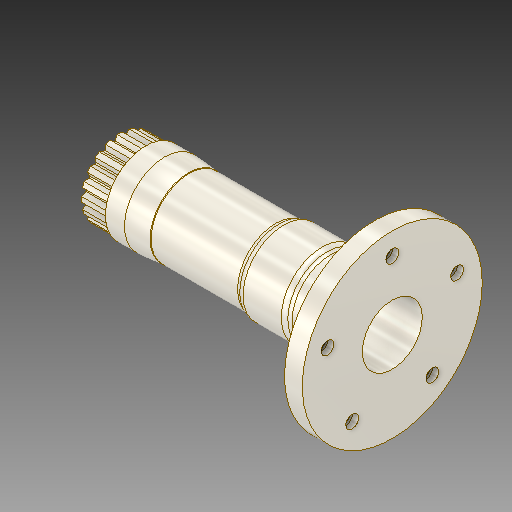
# Autodesk Inventor part: 301-04
Saved by Autodesk Inventor 2019 (Build 230136000, 136)
## iProperties
Company: Autodesk Inc.
Created: 2017-03-16
Part Number: 301-04
Material: Titanium
Document SubType Name: Modeling
Designer: Autodesk Inc.
Density: 4.51 g/cm^3
Appearance: Titanium
Mass: 190.026 g
Surface Area: 234.594 cm^2
Volume: 42.1344 cm^3
Author: Inventor
Autodesk Inventor part; units mm, degrees
ref_plane "YZ Plane" through (0, 0, 0) normal (1, 0, 0) x (0, 1, 0)
ref_plane "XZ Plane" through (0, 0, 0) normal (0, 1, 0) x (-1, 0, 0)
ref_plane "XY Plane" through (0, 0, 0) normal (0, 0, 1) x (1, 0, 0)
sketch "Sketch1" plane through (0, 0, 0) normal (0, 0, 1) x (1, 0, 0)
  line L0 (-20, 0) -> (120, 0) projected
  line L1 (0, 11) -> (100, 11)
  line L2 (0, 11) -> (0, 14.75)
  line L3 (0, 14.75) -> (16.5, 14.75)
  line L4 (58, 15) -> (76.5, 15)
  line L5 (76.5, 15) -> (76.5, 14)
  line L6 (25.3424, 14) -> (58, 14)
  line L7 (100, 14) -> (100, 11)
  line L8 (58, 14) -> (58, 15)
  line L9 (76.5, 14) -> (100, 14)
  arc A0 (25.3424, 14) -> (16.5, 14.75) centre (16.5, -37.75) ccw
  point P0 (0, 0)
  dimension "d0" = 100
  dimension "d1" = 22
  dimension "d2" = 3.75
  dimension "d3" = 16.5
  dimension "d9" = 3
  dimension "d10" = 52.5
  dimension "d11" = 58
  dimension "d12" = 18.5
  dimension "d13" = 4
  constraints: 18 end point, 4 parallel, 3 perpendicular, 2 point on circle, 2 vertical, 1 centre point, 1 collinear, 1 horizontal, 1 point on line, 1 tangent
  measures "d0" distance of L1.start L1.end
  measures "d1" diameter of L1 L0
  measures "d2" distance of L1.start L2.end
  measures "d3" distance of L2.end L3.end
  measures "d9" distance between parallel lines of L1 L6
  measures "d10" radius of A0
  measures "d11" distance between parallel lines of L2 L8
  measures "d12" distance between parallel lines of L8 L5
  measures "d13" distance between parallel lines of L1 L4
revolve "Revolution1" add sketch "Sketch1" angle 360 about axis through (-10, 0, 0) along (1, 0, 0)
fillet "Fillet1" radius 3 2 edges at (58, -15, 0) (76.5, -15, 0)
sketch "Sketch2" plane through (100, 0, 0) normal (1, 0, 0) x (0, 0, -1)
  circle A0 centre (0, 0) radius 14 projected
  circle A1 centre (0, 0) radius 11 projected
  circle A2 centre (0, 0) radius 33
  dimension "d17" = 66
  constraints: 1 centre point, 1 coincident
  measures "d17" diameter of A2
extrude "Extrusion1" add sketch "Sketch2" against normal blind 6.5 contours A2
fillet "Fillet2" radius 2 4 edges at (25.3424, -14, 0) (58, -14, 0) (76.5, -14, 0) (93.5, -14, 0)
ref_plane "Work Plane1" through (94.55, 0, 0) normal (-1, 0, 0) x (0, 0, 1)
sketch "Sketch3" plane through (94.55, 0, 0) normal (-1, 0, 0) x (0, 0, 1)
  circle A0 centre (0, 0) radius 33 projected
  point P0 (0, 25)
  dimension "d20" = 25
  constraints: 1 vertical alignment
  measures "d20" distance of A0.centre point (0, 25)
hole "Hole1" at (94.55, 25, 0) direction (1, 0, 0) diameter 6 depth 5 tip angle 110 start extended yes countersink diameter 11.4 countersink angle 90
pattern_circular "Circular Pattern1" count 5 over 360 about axis through (-10, 0, 0) along (1, 0, 0) of "Hole1"
sketch "Sketch4" plane through (0, 0, 0) normal (-1, 0, 0) x (0, 0, 1)
  circle A0 centre (0, 0) radius 11 projected
  circle A1 centre (0, 0) radius 14.75 projected
  arc A2 (-5.4322, 11.258) -> (-5.9149, 11.012) centre (0, 0) ccw
  line L0 (0, -21) -> (0, 21) construction
  line L1 (-0.9, 14) -> (0.9, 14)
  line L2 (-0.9, 14) -> (-1.6874, 12.3856)
  line L3 (0.9, 14) -> (1.6874, 12.3856)
  line L4 (-5.1822, 13.0367) -> (-5.4322, 11.258)
  line L5 (-5.1822, 13.0367) -> (-3.4703, 13.5929)
  line L6 (-3.4703, 13.5929) -> (-2.2225, 12.3008)
  line L7 (-8.9571, 10.7972) -> (-8.6452, 9.0283)
  line L8 (-8.9571, 10.7972) -> (-7.5009, 11.8552)
  line L9 (-7.5009, 11.8552) -> (-5.9149, 11.012)
  line L10 (-11.8552, 7.5009) -> (-11.012, 5.9149)
  line L11 (-11.8552, 7.5009) -> (-10.7972, 8.9571)
  line L12 (-10.7972, 8.9571) -> (-9.0283, 8.6452)
  line L13 (-13.5929, 3.4703) -> (-12.3008, 2.2225)
  line L14 (-13.5929, 3.4703) -> (-13.0367, 5.1822)
  line L15 (-13.0367, 5.1822) -> (-11.258, 5.4322)
  line L16 (-14, -0.9) -> (-12.3856, -1.6874)
  line L17 (-14, -0.9) -> (-14, 0.9)
  line L18 (-14, 0.9) -> (-12.3856, 1.6874)
  line L19 (-13.0367, -5.1822) -> (-11.258, -5.4322)
  line L20 (-13.0367, -5.1822) -> (-13.5929, -3.4703)
  line L21 (-13.5929, -3.4703) -> (-12.3008, -2.2225)
  line L22 (-10.7972, -8.9571) -> (-9.0283, -8.6452)
  line L23 (-10.7972, -8.9571) -> (-11.8552, -7.5009)
  line L24 (-11.8552, -7.5009) -> (-11.012, -5.9149)
  line L25 (-7.5009, -11.8552) -> (-5.9149, -11.012)
  line L26 (-7.5009, -11.8552) -> (-8.9571, -10.7972)
  line L27 (-8.9571, -10.7972) -> (-8.6452, -9.0283)
  line L28 (-3.4703, -13.5929) -> (-2.2225, -12.3008)
  line L29 (-3.4703, -13.5929) -> (-5.1822, -13.0367)
  line L30 (-5.1822, -13.0367) -> (-5.4322, -11.258)
  line L31 (0.9, -14) -> (1.6874, -12.3856)
  line L32 (0.9, -14) -> (-0.9, -14)
  line L33 (-0.9, -14) -> (-1.6874, -12.3856)
  line L34 (5.1822, -13.0367) -> (5.4322, -11.258)
  line L35 (5.1822, -13.0367) -> (3.4703, -13.5929)
  line L36 (3.4703, -13.5929) -> (2.2225, -12.3008)
  line L37 (8.9571, -10.7972) -> (8.6452, -9.0283)
  line L38 (8.9571, -10.7972) -> (7.5009, -11.8552)
  line L39 (7.5009, -11.8552) -> (5.9149, -11.012)
  line L40 (11.8552, -7.5009) -> (11.012, -5.9149)
  line L41 (11.8552, -7.5009) -> (10.7972, -8.9571)
  line L42 (10.7972, -8.9571) -> (9.0283, -8.6452)
  line L43 (13.5929, -3.4703) -> (12.3008, -2.2225)
  line L44 (13.5929, -3.4703) -> (13.0367, -5.1822)
  line L45 (13.0367, -5.1822) -> (11.258, -5.4322)
  line L46 (14, 0.9) -> (12.3856, 1.6874)
  line L47 (14, 0.9) -> (14, -0.9)
  line L48 (14, -0.9) -> (12.3856, -1.6874)
  line L49 (13.0367, 5.1822) -> (11.258, 5.4322)
  line L50 (13.0367, 5.1822) -> (13.5929, 3.4703)
  line L51 (13.5929, 3.4703) -> (12.3008, 2.2225)
  line L52 (10.7972, 8.9571) -> (9.0283, 8.6452)
  line L53 (10.7972, 8.9571) -> (11.8552, 7.5009)
  line L54 (11.8552, 7.5009) -> (11.012, 5.9149)
  line L55 (7.5009, 11.8552) -> (5.9149, 11.012)
  line L56 (7.5009, 11.8552) -> (8.9571, 10.7972)
  line L57 (8.9571, 10.7972) -> (8.6452, 9.0283)
  line L58 (3.4703, 13.5929) -> (2.2225, 12.3008)
  line L59 (3.4703, 13.5929) -> (5.1822, 13.0367)
  line L60 (5.1822, 13.0367) -> (5.4322, 11.258)
  arc A3 (-2.2225, 12.3008) -> (-5.4322, 11.258) centre (0, 0) ccw
  arc A4 (-5.9149, 11.012) -> (-8.6452, 9.0283) centre (0, 0) ccw
  arc A5 (-8.6452, 9.0283) -> (-9.0283, 8.6452) centre (0, 0) ccw
  arc A6 (-9.0283, 8.6452) -> (-11.012, 5.9149) centre (0, 0) ccw
  arc A7 (-11.012, 5.9149) -> (-11.258, 5.4322) centre (0, 0) ccw
  arc A8 (-11.258, 5.4322) -> (-12.3008, 2.2225) centre (0, 0) ccw
  arc A9 (-12.3008, 2.2225) -> (-12.3856, 1.6874) centre (0, 0) ccw
  arc A10 (-12.3856, 1.6874) -> (-12.3856, -1.6874) centre (0, 0) ccw
  arc A11 (-12.3856, -1.6874) -> (-12.3008, -2.2225) centre (0, 0) ccw
  arc A12 (-12.3008, -2.2225) -> (-11.258, -5.4322) centre (0, 0) ccw
  arc A13 (-11.258, -5.4322) -> (-11.012, -5.9149) centre (0, 0) ccw
  arc A14 (-11.012, -5.9149) -> (-9.0283, -8.6452) centre (0, 0) ccw
  arc A15 (-8.6452, -9.0283) -> (-5.9149, -11.012) centre (0, 0) ccw
  arc A16 (-5.9149, -11.012) -> (-5.4322, -11.258) centre (0, 0) ccw
  arc A17 (-5.4322, -11.258) -> (-2.2225, -12.3008) centre (0, 0) ccw
  arc A18 (-2.2225, -12.3008) -> (-1.6874, -12.3856) centre (0, 0) ccw
  arc A19 (-1.6874, -12.3856) -> (1.6874, -12.3856) centre (0, 0) ccw
  arc A20 (1.6874, -12.3856) -> (2.2225, -12.3008) centre (0, 0) ccw
  arc A21 (2.2225, -12.3008) -> (5.4322, -11.258) centre (0, 0) ccw
  arc A22 (5.4322, -11.258) -> (5.9149, -11.012) centre (0, 0) ccw
  arc A23 (5.9149, -11.012) -> (8.6452, -9.0283) centre (0, 0) ccw
  arc A24 (8.6452, -9.0283) -> (9.0283, -8.6452) centre (0, 0) ccw
  arc A25 (9.0283, -8.6452) -> (11.012, -5.9149) centre (0, 0) ccw
  arc A26 (11.012, -5.9149) -> (11.258, -5.4322) centre (0, 0) ccw
  arc A27 (11.258, -5.4322) -> (12.3008, -2.2225) centre (0, 0) ccw
  arc A28 (12.3008, -2.2225) -> (12.3856, -1.6874) centre (0, 0) ccw
  arc A29 (12.3856, -1.6874) -> (12.3856, 1.6874) centre (0, 0) ccw
  arc A30 (12.3856, 1.6874) -> (12.3008, 2.2225) centre (0, 0) ccw
  arc A31 (11.258, 5.4322) -> (11.012, 5.9149) centre (0, 0) ccw
  arc A32 (12.3008, 2.2225) -> (11.258, 5.4322) centre (0, 0) ccw
  arc A33 (11.012, 5.9149) -> (9.0283, 8.6452) centre (0, 0) ccw
  arc A34 (9.0283, 8.6452) -> (8.6452, 9.0283) centre (0, 0) ccw
  arc A35 (5.9149, 11.012) -> (5.4322, 11.258) centre (0, 0) ccw
  arc A36 (8.6452, 9.0283) -> (5.9149, 11.012) centre (0, 0) ccw
  arc A37 (2.2225, 12.3008) -> (1.6874, 12.3856) centre (0, 0) ccw
  arc A38 (5.4322, 11.258) -> (2.2225, 12.3008) centre (0, 0) ccw
  arc A39 (1.6874, 12.3856) -> (-1.6874, 12.3856) centre (0, 0) ccw
  arc A40 (-1.6874, 12.3856) -> (-2.2225, 12.3008) centre (0, 0) ccw
  arc A41 (-9.0283, -8.6452) -> (-8.6452, -9.0283) centre (0, 0) ccw
  point P0 (0, 14)
  point P1 (-4.3262, 13.3148)
  point P2 (-8.229, 11.3262)
  point P3 (-11.3262, 8.229)
  point P4 (-13.3148, 4.3262)
  point P5 (-14, 0)
  point P6 (-13.3148, -4.3262)
  point P7 (-11.3262, -8.229)
  point P8 (-8.229, -11.3262)
  point P9 (-4.3262, -13.3148)
  point P10 (0, -14)
  point P11 (4.3262, -13.3148)
  point P12 (8.229, -11.3262)
  point P13 (11.3262, -8.229)
  point P14 (13.3148, -4.3262)
  point P15 (14, 0)
  point P16 (13.3148, 4.3262)
  point P17 (11.3262, 8.229)
  point P18 (8.229, 11.3262)
  point P19 (4.3262, 13.3148)
  dimension "d32" = 25
  dimension "d33" = 1.8
  dimension "d34" = 14
  dimension "d35" = 116
  dimension "d38" = 360
  constraints: 118 end point, 2 vertical alignment, 1 horizontal, 1 horizontal alignment, 1 midpoint, 1 point on line, 279 other
  measures "d33" distance of L1.start L1.end
  measures "d34" distance from line of A0.centre L1
  measures "d35" angle of L1 L2
extrude "Extrusion2" cut sketch "Sketch4" against normal blind 9.5 contours A1
body "Solid1"
